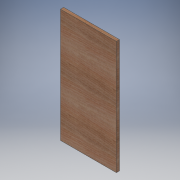
# Autodesk Inventor part: FrenteChico
Saved by Autodesk Inventor 2016 (Build 200138000, 138)
## iProperties
Created: 2018-06-25
Part Number: FrenteChico
Material: Wood (Birch)
Document SubType Name: Modeling
Designer: damia
Density: 0.55 g/cm^3
Appearance: Birch - Natural Polished
Mass: 2062.37 g
Surface Area: 4515.96 cm^2
Volume: 3749.76 cm^3
Author: damia
Autodesk Inventor part; units mm, degrees
ref_plane "YZ Plane" through (0, 0, 0) normal (1, 0, 0) x (0, 1, 0)
ref_plane "XZ Plane" through (0, 0, 0) normal (0, 1, 0) x (-1, 0, 0)
ref_plane "XY Plane" through (0, 0, 0) normal (0, 0, 1) x (1, 0, 0)
sketch "Sketch3" plane through (0, 0, 0) normal (0, 1, 0) x (-1, 0, 0)
  line L0 (0, 0) -> (-320, 0)
  line L1 (-320, 0) -> (-320, -651)
  line L2 (-320, -651) -> (0, -651)
  line L3 (0, -651) -> (0, 0)
  dimension "d13" = 320
  dimension "d14" = 651
  constraints: 8 end point, 2 parallel, 1 horizontal, 1 perpendicular
  measures "d13" distance of L2.end L1.end
  measures "d14" distance of L1.end L0.end
extrude "Extrusion3" add sketch "Sketch3" along normal blind 18
equation "\"d14\" = Profundidad"
equation "\"Profundidad\" = 651"
body "Solid2"
